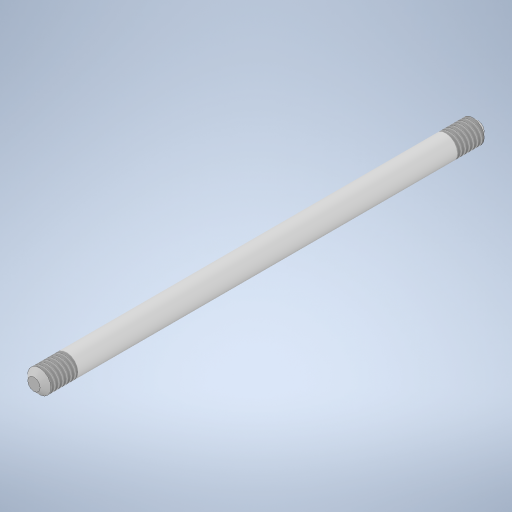
# Autodesk Inventor part: ES117_Axis
Saved by Autodesk Inventor 2024 (Build 280153000, 153)
## iProperties
Created: 2023-06-05
Part Number: ES117_Axis
Material: Generic
Document SubType Name: Modeling
Designer: vilas
Density: 1 g/cm^3
Appearance: Default
Author: vilas
Autodesk Inventor part; units mm, degrees
ref_plane "YZ Plane" through (0, 0, 0) normal (1, 0, 0) x (0, 1, 0)
ref_plane "XZ Plane" through (0, 0, 0) normal (0, 1, 0) x (-1, 0, 0)
ref_plane "XY Plane" through (0, 0, 0) normal (0, 0, 1) x (1, 0, 0)
sketch "Sketch1" plane through (0, 0, 0) normal (0, 0, 1) x (1, 0, 0)
  circle A0 centre (0, 0) radius 2.15
  dimension "d0" = 4.3
  constraints: 1 centre point, 1 coincident
  measures "d0" diameter of A0
extrude "Extrusion1" add sketch "Sketch1" along normal mid plane 82
chamfer "Chamfer1" distance 1 angle 45 2 edges at (-2.15, 0, 41) (-2.15, 0, -41)
thread "Thread1" size "M4.5x0.75" class "6g" standard "ISO Metric profile" length 5
thread "Thread2" size "M4.5x0.75" class "6g" standard "ANSI Metric M Profile" length 5
body "Solid1"
